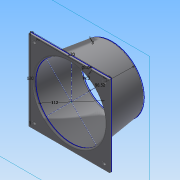
# Autodesk Inventor part: 120mm-4in duct adapter
Saved by Autodesk Inventor 2014 SP2 (Build 180246200, 246)
## iProperties
Created: 2014-07-18
Part Number: 120mm-4in duct adapter
Material: Generic
Document SubType Name: Modeling
Designer: dliu
Density: 1 g/cm^3
Appearance: Default
Author: dliu
Autodesk Inventor part; units mm, degrees
ref_plane "YZ Plane" through (0, 0, 0) normal (1, 0, 0) x (0, 1, 0)
ref_plane "XY Plane" through (0, 0, 0) normal (0, 0, 1) x (1, 0, 0)
sketch "Sketch1" plane through (0, 0, 0) normal (0, 1, 0) x (-1, 0, 0)
  line L0 (-60, -60) -> (60, -60)
  line L1 (60, -60) -> (60, 60)
  line L2 (60, 60) -> (-60, 60)
  line L3 (-60, 60) -> (-60, -60)
  line L4 (-60, -60) -> (60, 60) construction
  line L5 (60, -60) -> (-60, 60) construction
  circle A0 centre (0, 0) radius 56
  line L6 (0, 60) -> (0, 0) construction
  circle A1 centre (0, 0) radius 53
  point P0 (-52, 52)
  dimension "d0" = 120
  dimension "d1" = 120
  dimension "d2" = 112
  dimension "d4" = 104
  dimension "d29" = 3
  constraints: 14 end point, 3 midpoint, 3 parallel, 2 centre point, 1 coincident, 1 horizontal, 1 perpendicular, 1 point on line
  measures "d0" distance of L2.end L1.end
  measures "d1" distance of L1.end L0.end
  measures "d2" diameter of A0
  measures "d4" diameter of point (-52, 52) L6
  measures "d29" radial gap between concentric circles of A0 A1
extrude "Extrusion1" add sketch "Sketch1" against normal blind 3 contours L3 L2 L1 L0 | A0
hole "Hole1" at (52, 0, 52) direction (0, -1, 0) diameter 4.4 end through all
pattern_circular "Circular Pattern1" count 4 over 360 about axis through (0, -10, 0) along (0, 1, 0) of "Hole1"
ref_plane "Work Plane1" through (0, 60, 0) normal (0, 1, 0) x (-1, 0, 0)
sketch "Sketch3" plane through (0, 60, 0) normal (0, 1, 0) x (-1, 0, 0)
  circle A0 centre (0, 0) radius 48.26
  circle A1 centre (0, 0) radius 45.26
  dimension "d21" = 96.52
  dimension "WallThickness" = 3
  constraints: 2 centre point, 1 coincident
  measures "d21" diameter of A0
  measures "WallThickness" radial gap between concentric circles of A0 A1
loft "Loft1" add profiles "Sketch3", "Sketch1" contours A0 | A1 / A0 | A1
loft "Loft2" cut profiles "Sketch1", "Sketch3" contours A1 / A1
fillet "Fillet1" radius 2 3 edges at (56, 0, 0) (53, 0, 0) (53, -3, 0)
fillet "Fillet2" radius 1.5 2 edges at (48.26, 60, 0) (45.26, 60, 0)
equation "\"d29\" = WallThickness"
equation "\"d36\" = 0.5 * WallThickness"
body "Solid1"
